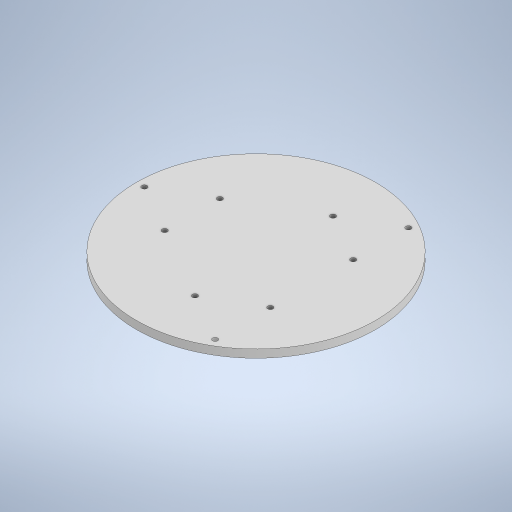
# Autodesk Inventor part: base_frame_3
Saved by Autodesk Inventor 2023.1 (Build 271208000, 208)
## iProperties
Created: 2023-11-14
Part Number: base_frame_3
Material: Generic
Document SubType Name: Modeling
Designer: zavrel
Density: 1 g/cm^3
Appearance: Default
Author: zavrel
Autodesk Inventor part; units mm, degrees
ref_plane "YZ Plane" through (0, 0, 0) normal (1, 0, 0) x (0, 1, 0)
ref_plane "XZ Plane" through (0, 0, 0) normal (0, 1, 0) x (-1, 0, 0)
ref_plane "XY Plane" through (0, 0, 0) normal (0, 0, 1) x (1, 0, 0)
sketch "Sketch1" plane through (0, 0, 0) normal (0, 1, 0) x (-1, 0, 0)
  circle A0 centre (0, 0) radius 75
  dimension "d0" = 150
  constraints: 1 centre point, 1 coincident
  measures "d0" diameter of A0
extrude "Extrusion1" add sketch "Sketch1" along normal blind 5
sketch "Sketch2" plane through (0, 5, 0) normal (0, 1, 0) x (1, 0, 0)
  circle A0 centre (0, 0) radius 75 projected
  circle A1 centre (0, 0) radius 50 construction
  circle A2 centre (-50, 0) radius 20 construction
  circle A3 centre (-70, 0) radius 1.6
  circle A4 centre (-40, -17.3205) radius 1.6
  circle A5 centre (-40, 17.3205) radius 1.6
  circle A6 centre (25, -43.3013) radius 20 construction
  circle A7 centre (35, -60.6218) radius 1.6
  circle A8 centre (35, -25.9808) radius 1.6
  circle A9 centre (5, -43.3013) radius 1.6
  circle A10 centre (25, 43.3013) radius 20 construction
  circle A11 centre (35, 60.6218) radius 1.6
  circle A12 centre (5, 43.3013) radius 1.6
  circle A13 centre (35, 25.9808) radius 1.6
  dimension "d3" = 100
  dimension "d4" = 40
  dimension "d5" = 3.2
  dimension "d8" = 360
  dimension "d12" = 360
  constraints: 9 centre point, 2 horizontal alignment, 1 coincident, 42 other
  measures "d5" diameter of A3
extrude "Extrusion2" cut sketch "Sketch2" against normal through all contours A3 | A4 | A5 | A7 | A8 | A9 | A11 | A12 | A13
body "Solid1"
